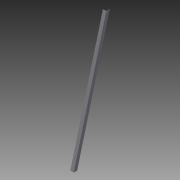
# Autodesk Inventor part: Front Left Beam
Saved by Autodesk Inventor 2015 (Build 190159000, 159)
## iProperties
Created: 2015-01-10
Part Number: Front Left Beam
Material: Generic
Document SubType Name: Modeling
Designer: Chandler Willoughby
Density: 1 g/cm^3
Appearance: Default
Author: Chandler Willoughby
Autodesk Inventor part; units mm, degrees
ref_plane "YZ Plane" through (0, 0, 0) normal (1, 0, 0) x (0, 1, 0)
ref_plane "XZ Plane" through (0, 0, 0) normal (0, 1, 0) x (-1, 0, 0)
ref_plane "XY Plane" through (0, 0, 0) normal (0, 0, 1) x (1, 0, 0)
sketch "Sketch1" plane through (0, 0, 0) normal (1, 0, 0) x (0, 1, 0)
  line L0 (1828.8, -482.6) -> (0, 0)
  line L1 (1828.8, -482.6) -> (1828.8, -533.4)
  line L2 (0, 0) -> (0, -50.8)
  line L3 (0, -50.8) -> (1828.8, -533.4)
  dimension "d3" = 50.8
  dimension "d4" = 50.8
  constraints: 8 end point, 2 vertical
  measures "d3" distance of L0.start L1.end
  measures "d4" distance of L0.end L2.end
extrude "Extrusion1" add sketch "Sketch1" along normal blind 3.175
sketch "Sketch2" plane through (0, 0, 0) normal (-1, 0, 0) x (0, 0, 1)
  line L0 (0, 0) -> (-482.6, 1828.8)
  line L1 (-482.6, 1828.8) -> (0, 0) projected
  line L2 (-482.6, 1828.8) -> (-485.775, 1828.8)
  line L3 (-533.4, 1828.8) -> (-482.6, 1828.8) projected
  line L4 (0, 0) -> (-3.175, 0)
  line L5 (0, 0) -> (-50.8, 0) projected
  line L6 (-50.8, 0) -> (-533.4, 1828.8) projected
  line L7 (-3.175, 0) -> (-485.775, 1828.8)
  dimension "d7" = 3.175
  dimension "d8" = 3.175
  constraints: 8 end point, 2 point on line, 1 collinear
  measures "d7" distance of L0.end L2.end
  measures "d8" distance of L0.start L4.end
extrude "Extrusion2" add sketch "Sketch2" along normal blind 47.625 contours L4 L7 L2 L0
body "Solid1"
